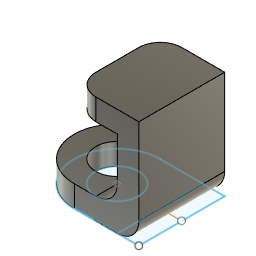
Exercise3 (Autodesk Fusion 360 design; units mm, degrees)
Autodesk Fusion 360 part; units mm, degrees
sketch "Sketch1" plane through (0, 0, 0) normal (0, 0, 1) x (1, 0, 0) in component "Exercise3"
  circle A0 centre (0, 0) radius 10
  line L0 (0, 0) -> (30, 0) construction
  line L1 (0.1031, 19.9997) -> (30.1031, 19.9997)
  line L2 (0.1031, -19.9997) -> (30.1031, -19.9997)
  line L3 (30.1031, 19.9997) -> (30.1031, -20.0003)
  arc A1 (0.1031, 19.9997) -> (0.1031, -19.9997) centre (0, 0) ccw
  line L4 (20.1031, 19.9997) -> (20.1031, -19.9997)
  dimension "d1" = 20
  dimension "d2" = 40
  dimension "d3" = 30
  dimension "d4" = 30
  dimension "d5" = 30
  dimension "d6" = 40
  dimension "d7" = 10
  constraint coincident A0.centre L0.start
  constraint horizontal L0
  constraint horizontal L1
  constraint parallel L0 L2
  constraint perpendicular L2 L3
  constraint symmetric L0 L1 L2
  constraint coincident L1 L4.start
  constraint coincident L2 L4.end
  constraint perpendicular L2 L4
  measures "d1" diameter of A0
  measures "d2" diameter of A1
  measures "d3" distance of A0.centre L0.end
  measures "d4" distance of L1.start L1.end
  measures "d5" distance of L2.start L2.end
  measures "d6" distance of L1.end L3.end
  measures "d7" distance of L3 L4
extrude "Extrude1" add sketch "Sketch1" along normal blind 10 contours L1 L2 A1 L4 in component "Exercise3"
extrude "Extrude2" add sketch "Sketch1" along normal blind 50.06 contours L1 L2 L3 L4 in component "Exercise3"
fillet "Fillet1" radius 10 1 edges at (30.1031, 0, 0) in component "Exercise3"
sketch "Sketch2" plane through (0, 0, 50.06) normal (0, 0, 1) x (-1, 0, 0) in component "Exercise3"
  line L0 (-30.1031, -19.9997) -> (-20.1031, -19.9997)
  line L1 (-20.1031, -19.9997) -> (-20.1031, 19.9997)
  line L2 (-20.1031, 19.9997) -> (-30.1031, 19.9997)
  line L3 (-30.1031, 19.9997) -> (-30.1031, -19.9997)
  line L4 (-30.1031, 0) -> (0, 0) construction
  line L5 (-30.1031, -19.9997) -> (-0.1031, -19.9997)
  line L6 (-0.1031, -19.9997) -> (-0.1031, 19.9997)
  line L7 (-0.1031, 19.9997) -> (-30.1031, 19.9997)
  line L8 (-30.1031, 19.9997) -> (-30.1031, -19.9997)
  dimension "d13" = 30
  constraint midpoint L3 L4.start
  constraint coincident L4.end origin
  constraint horizontal L5
  constraint vertical L6
  constraint horizontal L7
  constraint vertical L8
  constraint coincident L0.start L3.end
  constraint symmetric L4 L5 L7
  measures "d13" distance of L6 L8
extrude "Extrude3" add sketch "Sketch2" against normal blind 10 contours L1 L5 L6 L7 in component "Exercise3"
fillet "Fillet2" radius 10 2 edges at (0.1031, -19.9997, 45.06) (0.1031, 19.9997, 45.06) in component "Exercise3"
fillet "Fillet3" radius 10 1 edges at (20.1031, 0, 10) in component "Exercise3"
component "Exercise3" placed x (1, 0, 0) y (0, 1, 0) z (0, 0, 1) at (0, 0, 0)
